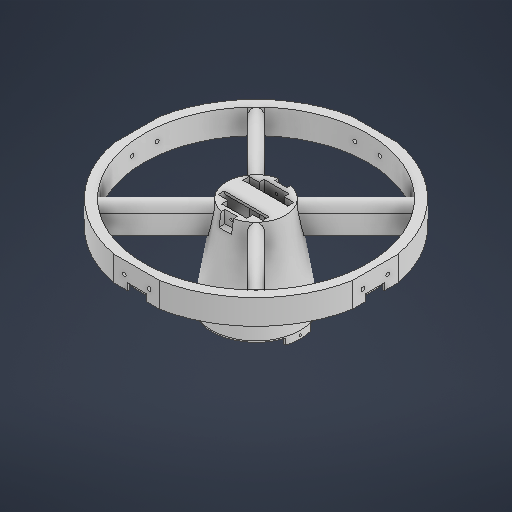
# Autodesk Inventor part: 004-002
Saved by Autodesk Inventor 2026 (Build 300175000, 175)
## iProperties
Created: 2026-04-19
Part Number: 004-002
Material: Ogólny
Document SubType Name: Modeling
Designer: Patryk Lombardo
Density: 1 g/cm^3
Appearance: Domyślna
Author: Patryk Lombardo
Autodesk Inventor part; units mm, degrees
ref_plane "YZ Plane" through (0, 0, 0) normal (1, 0, 0) x (0, 1, 0)
ref_plane "XZ Plane" through (0, 0, 0) normal (0, 1, 0) x (-1, 0, 0)
sketch "Szkic1" plane through (0, 0, 0) normal (0, 1, 0) x (-1, 0, 0)
  circle A0 centre (0, 0) radius 35.5
  dimension "d0" = 71
  constraints: 1 centre point, 1 coincident
  measures "d0" diameter of A0
extrude "Wyciągnięcie proste1" add sketch "Szkic1" against normal blind 1
ref_plane "Płaszczyzna konstrukcyjna1" through (0, 74, 0) normal (0, 1, 0) x (1, 0, 0)
sketch "Szkic2" plane through (0, 74, 0) normal (0, 1, 0) x (1, 0, 0)
  circle A0 centre (0, 0) radius 23.5
  line L0 (-18, 0) -> (18, 0) construction
  line L1 (0, -12.5) -> (0, 12.5) construction
  line L2 (18, 12.5) -> (18, -12.5) construction
  line L3 (-18, 12.5) -> (-18, -12.5) construction
  line L4 (-18, 12.5) -> (18, 12.5) construction
  line L5 (-18, -12.5) -> (18, -12.5) construction
  dimension "d4" = 47
  dimension "d5" = 36
  dimension "d6" = 25
  dimension "d7" = 12.5
  constraints: 12 end point, 4 midpoint, 3 vertical, 2 horizontal, 1 centre point, 1 coincident, 1 parallel
  measures "d4" diameter of A0
  measures "d5" distance of L0.start L0.end
  measures "d6" distance of L1.start L1.end
  measures "d7" distance between parallel lines of L4 L0
loft "Wyciągnięcie złożone1" add profiles "Szkic2" section 1 edges at (35.5, 0, 0)
sketch "Szkic3" plane through (0, 74, 0) normal (0, 1, 0) x (1, 0, 0)
  line L0 (-18, 0) -> (18, 0) construction
  line L1 (0, 12.5) -> (0, -12.5) construction
  line L2 (18, 12.5) -> (18, -12.5)
  line L3 (-18, 12.5) -> (-18, -12.5)
  line L4 (-18, 12.5) -> (18, 12.5)
  line L5 (-18, -12.5) -> (18, -12.5)
  line L6 (0, 12.5) -> (0, 16.5) construction
  line L7 (10, 16.5) -> (-10, 16.5)
  line L8 (-10, 16.5) -> (-10, 12.5)
  line L9 (10, 16.5) -> (10, 12.5)
  line L10 (0, -12.5) -> (0, -17.5) construction
  line L11 (-10, -17.5) -> (10, -17.5)
  line L12 (-10, -17.5) -> (-10, -12.5)
  line L13 (10, -17.5) -> (10, -12.5)
  point P0 (0, 0)
  dimension "d12" = 36
  dimension "d13" = 25
  dimension "d14" = 12.5
  dimension "d15" = 4
  dimension "d16" = 20
  dimension "d17" = 5
  dimension "d18" = 20
  constraints: 28 end point, 6 midpoint, 6 vertical, 4 perpendicular, 4 point on line, 3 horizontal, 1 parallel
  measures "d12" distance of L0.start L0.end
  measures "d13" distance of L1.start L1.end
  measures "d14" distance between parallel lines of L4 L0
  measures "d15" distance of L1.start L6.end
  measures "d16" distance of L7.start L7.end
  measures "d17" distance of L1.end L10.end
  measures "d18" distance of L11.start L11.end
extrude "Wyciągnięcie proste2" cut sketch "Szkic3" against normal through all
sketch "Szkic4" plane through (0, 74, 0) normal (0, 1, 0) x (1, 0, 0)
  line L0 (18, 0) -> (-18, 0) construction
  line L1 (-18, -7.5) -> (-18, 7.5)
  line L2 (18, -7.5) -> (18, 7.5)
  line L3 (-18, 7.5) -> (18, 7.5)
  line L4 (-18, -7.5) -> (18, -7.5)
  point P0 (0, 0)
  dimension "d21" = 36
  dimension "d22" = 15
  constraints: 10 end point, 3 midpoint, 2 horizontal, 2 vertical, 1 parallel
  measures "d21" distance of L0.start L0.end
  measures "d22" distance of L1.start L1.end
extrude "Wyciągnięcie proste3" add sketch "Szkic4" against normal blind 2
sketch "Szkic6" plane through (0, -1, 0) normal (0, -1, 0) x (1, 0, 0)
  line L0 (-19.5, 0) -> (19.5, 0) construction
  line L1 (0, 14) -> (0, -14) construction
  line L2 (19.5, 14.5) -> (19.5, -14.5)
  line L3 (-19.5, 14.5) -> (-19.5, -14.5)
  line L4 (-19.5, 14.5) -> (19.5, 14.5)
  line L5 (-19.5, -14.5) -> (19.5, -14.5)
  line L6 (0, 14) -> (0, 19) construction
  line L7 (12, 19) -> (-12, 19)
  line L8 (-12, 19) -> (-12, 14.5)
  line L9 (12, 19) -> (12, 14.5)
  line L10 (0, -14) -> (0, -19) construction
  line L11 (-12, -19) -> (12, -19)
  line L12 (-12, -19) -> (-12, -14.5)
  line L13 (12, -19) -> (12, -14.5)
  circle A0 centre (0, 0) radius 31
  dimension "d25" = 39
  dimension "d26" = 28
  dimension "d27" = 14.5
  dimension "d28" = 5
  dimension "d29" = 24
  dimension "d30" = 5
  dimension "d31" = 24
  dimension "d32" = 62
  constraints: 28 end point, 6 midpoint, 6 vertical, 4 perpendicular, 4 point on line, 3 horizontal, 2 coincident, 1 centre point, 1 parallel
  measures "d25" distance of L0.start L0.end
  measures "d26" distance of L1.start L1.end
  measures "d27" distance between parallel lines of L4 L0
  measures "d28" distance of L1.start L6.end
  measures "d29" distance of L7.start L7.end
  measures "d30" distance of L1.end L10.end
  measures "d31" distance of L11.start L11.end
  measures "d32" diameter of A0
extrude "Wyciągnięcie proste4" cut sketch "Szkic6" against normal blind 18
sketch "Szkic7" plane through (0, -1, 0) normal (0, -1, 0) x (1, 0, 0)
  line L0 (32, 0) -> (-32, 0) construction
  circle A0 centre (0, 0) radius 35.5
  line L1 (-32, -10) -> (-32, 10)
  line L2 (32, -10) -> (32, 10)
  line L3 (32, -10) -> (34.0624, -10)
  line L4 (32, 10) -> (34.0624, 10)
  line L5 (-32, -10) -> (-34.0624, -10)
  line L6 (-32, 10) -> (-34.0624, 10)
  dimension "d35" = 64
  dimension "d36" = 71
  dimension "d37" = 20
  dimension "d38" = 20
  constraints: 14 end point, 4 coincident, 4 horizontal, 4 point on circle, 3 midpoint, 2 vertical, 1 centre point, 1 parallel
  measures "d35" distance of L0.start L0.end
  measures "d36" diameter of A0
  measures "d37" distance of L1.start L1.end
  measures "d38" distance of L2.start L2.end
extrude "Wyciągnięcie proste5" add sketch "Szkic7" along normal blind 5 contours A0 L3 L2 L4 | L6 L1 L5 A0
sketch "Szkic8" plane through (32, -1, -10) normal (-1, 0, 0) x (0, 0, 1)
  line L0 (10, 1) -> (10, -2.5) construction
  circle A0 centre (10, -2.5) radius 1
  dimension "d41" = 3.5
  dimension "d42" = 2
  constraints: 2 end point, 1 centre point, 1 coincident, 1 vertical
  measures "d41" distance of L0.start L0.end
  measures "d42" diameter of A0
extrude "Wyciągnięcie proste6" cut sketch "Szkic8" along normal through all both and the other way through all
sketch "Szkic9" plane through (0, 74, 0) normal (0, 1, 0) x (1, 0, 0)
  circle A0 centre (0, 0) radius 23.5
  line L0 (0, -20) -> (0, 20) construction
  line L1 (-5, 20) -> (5, 20)
  line L2 (-5, -20) -> (5, -20)
  line L3 (5, 20) -> (5, 30)
  line L4 (5, -20) -> (5, -30)
  line L5 (-5, -20) -> (-5, -30)
  line L6 (-5, -30) -> (5, -30)
  line L7 (-5, 20) -> (-5, 30)
  line L8 (-5, 30) -> (5, 30)
  dimension "d45" = 47
  dimension "d46" = 40
  dimension "d47" = 10
  dimension "d48" = 10
  dimension "d49" = 10
  dimension "d50" = 10
  constraints: 18 end point, 4 vertical, 3 midpoint, 2 horizontal, 2 perpendicular, 1 centre point, 1 coincident, 1 point on line
  measures "d45" diameter of A0
  measures "d46" distance of L0.start L0.end
  measures "d47" distance of L2.start L2.end
  measures "d48" distance of L1.start L1.end
  measures "d49" distance of L1.end L3.end
  measures "d50" distance of L2.end L4.end
extrude "Wyciągnięcie proste7" cut sketch "Szkic9" against normal blind 10 contours L3 L1 L7 A0 | A0 L7 L8 L3 | L4 L6 L5 A0 | A0 L5 L2 L4
sketch "Szkic10" plane through (5, 74, -20) normal (0, 0, -1) x (-1, 0, 0)
  line L0 (0, 0) -> (5, 0) construction
  line L1 (5, 0) -> (5, -5) construction
  circle A0 centre (5, -5) radius 1
  point P0 (5, -74)
  dimension "d53" = 5
  dimension "d54" = 5
  dimension "d55" = 0
  dimension "d56" = 74
  dimension "d57" = 2
  constraints: 4 end point, 1 centre point, 1 coincident, 1 horizontal, 1 perpendicular
  measures "d53" distance of L0.start L0.end
  measures "d54" distance of L0.end L1.end
  measures "d55" distance from line of point (5, -74) L1
  measures "d56" distance from line of point (5, -74) L0
  measures "d57" diameter of A0
extrude "Wyciągnięcie proste8" cut sketch "Szkic10" against normal through all
sketch "Szkic11" plane through (-5, 74, 20) normal (0, 1, 0) x (1, 0, 0)
  circle A0 centre (5, 20) radius 90
  circle A1 centre (5, 20) radius 97.5
  line L0 (5, 20) -> (5, -75.75) construction
  line L1 (-13.3899, -75.75) -> (23.3899, -75.75)
  line L2 (5, 20) -> (100.75, 20) construction
  line L3 (100.75, 1.6101) -> (100.75, 38.3899)
  line L4 (5, 20) -> (5, 115.75) construction
  line L5 (23.3899, 115.75) -> (-13.3899, 115.75)
  line L6 (5, 20) -> (-90.75, 20) construction
  line L7 (-90.75, 38.3899) -> (-90.75, 1.6101)
  line L8 (5, 20) -> (68.6396, 83.6396) construction
  line L9 (64.9467, 87.1296) -> (72.1296, 79.9467)
  line L10 (5, 20) -> (-58.6396, 83.6396) construction
  line L11 (-62.1296, 79.9467) -> (-54.9467, 87.1296)
  line L12 (5, 20) -> (-58.6396, -43.6396) construction
  line L13 (-54.9467, -47.1296) -> (-62.1296, -39.9467)
  line L14 (5, 20) -> (68.6396, -43.6396) construction
  line L15 (72.1296, -39.9467) -> (64.9467, -47.1296)
  point P0 (-93.9108, 38.2483)
  point P1 (-93.9108, 1.4686)
  point P2 (-16.5506, -75.8915)
  point P3 (97.5892, 1.4686)
  point P4 (97.5892, 38.2483)
  point P5 (20.2291, 115.6085)
  point P6 (-16.5506, 115.6085)
  point P7 (68.5382, 83.5382)
  point P8 (-58.5382, 83.5382)
  point P9 (-58.5382, -43.5382)
  point P10 (68.5382, -43.5382)
  point P11 (-90.75, 1.6101)
  point P12 (-13.3899, -75.75)
  point P13 (-13.3899, 115.75)
  dimension "d63" = 195
  dimension "d62" = 180
  dimension "d64" = 95.75
  dimension "d65" = 360
  dimension "d66" = 45
  dimension "d67" = 10.1581
  dimension "d70" = 360
  constraints: 32 end point, 4 point on line, 3 coincident, 2 midpoint, 2 point on circle, 1 centre point, 1 horizontal, 1 perpendicular, 1 vertical, 57 other
  measures "d62" diameter of A0
  measures "d64" distance of L0.start L0.end
  measures "d66" angle of L4 L8
  measures "d67" distance of L9.start L9.end
extrude "Wyciągnięcie proste9" add sketch "Szkic11" against normal blind 20 contours L9 A0 | A0 L15 | L11 A0 | A0 L13 | L3 A1 L1 L7 L5
sketch "Szkic13" plane through (-5, 74, 20) normal (0, 1, 0) x (1, 0, 0)
  line L0 (5, 20) -> (5, 10) construction
  line L1 (5, 10) -> (5, 0) construction
  line L2 (5, 20) -> (5, 27) construction
  line L3 (10, 20) -> (0, 20) construction
  ellipse E0 centre (5, 20) end of major axis (0, 20) minor radius 7 (10, 20) -> (0, 20) ccw
  ellipse E1 centre (5, 20) end of major axis (0, 20) minor radius 20 (0, 20) -> (10, 20) ccw
  line L4 (2.25, 10) -> (7.75, 10)
  line L5 (7.75, 10) -> (7.75, 3.2967)
  line L6 (2.25, 10) -> (2.25, 3.2967)
  dimension "d80" = 10
  dimension "d81" = 7
  dimension "d82" = 10
  dimension "d83" = 10
  dimension "d84" = 5.5
  constraints: 14 end point, 4 horizontal, 4 vertical, 2 coincident, 2 midpoint, 1 point on line, 12 other
  measures "d80" distance of L3.end L3.start
  measures "d81" distance of L0.start L2.end
  measures "d82" distance of L0.end L1.end
  measures "d83" distance of L0.start L0.end
  measures "d84" distance of L4.start L4.end
sketch "Szkic14" plane through (59.9467, 54, -67.1296) normal (-0.7071068, 0, 0.7071068) x (0.7071068, 0, 0.7071068)
  line L0 (5.0791, 12.9138) -> (5.0791, 2.9138) construction
  line L1 (5.0791, 2.9138) -> (5.0791, -7.0862) construction
  line L2 (5.0791, 12.9138) -> (5.0791, 19.9138) construction
  line L3 (10.0791, 12.9138) -> (0.0791, 12.9138) construction
  ellipse E0 centre (5.0791, 12.9138) end of major axis (0.0791, 12.9138) minor radius 7 (10.0791, 12.9138) -> (0.0791, 12.9138) ccw
  ellipse E1 centre (5.0791, 12.9138) end of major axis (0.0791, 12.9138) minor radius 20 (0.0791, 12.9138) -> (10.0791, 12.9138) ccw
  line L4 (2.3291, 2.9138) -> (7.8291, 2.9138)
  line L5 (7.8291, 2.9138) -> (7.8291, -3.7895)
  line L6 (2.3291, 2.9138) -> (2.3291, -3.7895)
  point P0 (5.0791, -54)
  dimension "d85" = 10
  dimension "d86" = 7
  dimension "d87" = 10
  dimension "d88" = 10
  dimension "d89" = 5.5
  dimension "d90" = 2.75
  dimension "d91" = 66.9138
  constraints: 14 end point, 4 horizontal, 4 vertical, 2 coincident, 2 midpoint, 1 point on line, 12 other
  measures "d85" distance of L3.end L3.start
  measures "d86" distance of L0.start L2.end
  measures "d87" distance of L0.end L1.end
  measures "d88" distance of L0.start L0.end
  measures "d89" distance of L4.start L4.end
  measures "d90" distance from line of point (5.079, -54) L5
  measures "d91" distance from line of point (5.079, -54) L3
extrude "Wyciągnięcie proste10" add sketch "Szkic14" along normal up to surface contours E1 L5 L4 L6 E0
pattern_circular "Szyk kołowy1" count 4 over 360 about axis through (0, 0, 0) along (0, 1, 0) of "Wyciągnięcie proste10"
sketch "Szkic15" plane through (-5, 54, 20) normal (0, -1, 0) x (1, 0, 0)
  circle A0 centre (5, -20) radius 91.5
  circle A1 centre (5, -20) radius 94.5
  line L0 (5, -20) -> (-86.5, -20) construction
  line L1 (-86.5, -27.5) -> (-86.5, -12.5)
  line L2 (-86.5, -27.5) -> (-92.5, -27.5)
  line L3 (-92.5, -27.5) -> (-92.5, -12.5)
  line L4 (-92.5, -12.5) -> (-86.5, -12.5)
  line L5 (5, -20) -> (5, -111.5) construction
  line L6 (12.5, -111.5) -> (-2.5, -111.5)
  line L7 (12.5, -111.5) -> (12.5, -117.5)
  line L8 (12.5, -117.5) -> (-2.5, -117.5)
  line L9 (-2.5, -117.5) -> (-2.5, -111.5)
  line L10 (5, -20) -> (96.5, -20) construction
  line L11 (96.5, -12.5) -> (96.5, -27.5)
  line L12 (96.5, -12.5) -> (102.5, -12.5)
  line L13 (102.5, -12.5) -> (102.5, -27.5)
  line L14 (102.5, -27.5) -> (96.5, -27.5)
  line L15 (5, -20) -> (5, 71.5) construction
  line L16 (-2.5, 71.5) -> (12.5, 71.5)
  line L17 (-2.5, 71.5) -> (-2.5, 77.5)
  line L18 (-2.5, 77.5) -> (12.5, 77.5)
  line L19 (12.5, 77.5) -> (12.5, 71.5)
  circle A2 centre (5, -20) radius 35.5
  line L20 (5, -20) -> (-20.1023, -45.1023) construction
  line L21 (-2.955, -31.844) -> (-6.844, -27.955)
  line L22 (-6.844, -27.955) -> (-21.9714, -43.0823)
  line L23 (-2.955, -31.844) -> (-18.0823, -46.9714)
  line L24 (5, -20) -> (30.1023, -45.1023) construction
  line L25 (16.844, -27.955) -> (12.955, -31.844)
  line L26 (12.955, -31.844) -> (28.0823, -46.9714)
  line L27 (16.844, -27.955) -> (31.9714, -43.0823)
  line L28 (5, -20) -> (30.1023, 5.1023) construction
  line L29 (12.955, -8.156) -> (16.844, -12.045)
  line L30 (16.844, -12.045) -> (31.9714, 3.0823)
  line L31 (12.955, -8.156) -> (28.0823, 6.9714)
  line L32 (5, -20) -> (-20.1023, 5.1023) construction
  line L33 (-6.844, -12.045) -> (-2.955, -8.156)
  line L34 (-2.955, -8.156) -> (-18.0823, 6.9714)
  line L35 (-6.844, -12.045) -> (-21.9714, 3.0823)
  line L36 (-6.6295, -4.4814) -> (16.6295, -4.4814)
  line L37 (-6.6295, -35.5186) -> (16.6295, -35.5186)
  line L38 (-6.6295, -4.4814) -> (-6.6295, -35.5186)
  line L39 (16.6295, -4.4814) -> (16.6295, -35.5186)
  point P0 (-4.8995, -29.8995)
  point P1 (14.8995, -29.8995)
  point P2 (14.8995, -10.1005)
  point P3 (-4.8995, -10.1005)
  point P4 (-89.2019, -12.5)
  point P5 (-89.2019, -27.5)
  point P6 (-2.5, -114.2019)
  point P7 (12.5, -114.2019)
  point P8 (99.2019, -27.5)
  point P9 (99.2019, -12.5)
  point P10 (12.5, 74.2019)
  point P11 (-2.5, 74.2019)
  point P12 (-21.9714, 3.0823)
  point P13 (5, -4.4814)
  point P14 (16.6295, -28.1694)
  point P15 (16.6295, -11.8306)
  point P16 (-6.6295, -4.4814)
  point P17 (-6.6295, -11.8306)
  point P18 (-6.6295, -28.1694)
  dimension "d97" = 183
  dimension "d98" = 189
  dimension "d99" = 15
  dimension "d100" = 6
  dimension "d103" = 360
  dimension "d105" = 71
  dimension "d106" = 45
  dimension "d107" = 5.5
  dimension "d108" = 14
  dimension "d109" = 21.3933
  dimension "d112" = 360
  dimension "d116" = 23.2591
  dimension "d117" = 23.2591
  constraints: 80 end point, 8 point on line, 4 perpendicular, 3 coincident, 3 horizontal, 3 midpoint, 3 point on circle, 2 centre point, 2 vertical, 1 horizontal alignment, 1 parallel, 92 other
  measures "d98" diameter of A1
  measures "d99" distance of L1.start L1.end
  measures "d100" distance of L1.start L2.end
  measures "d105" diameter of A2
  measures "d106" angle of L5 L20
  measures "d107" distance of L21.start L21.end
  measures "d108" distance of point (-4.899, -29.899) point (5, -20)
  measures "d109" distance of L21.end L22.end
  measures "d116" distance of L37.start L37.end
  measures "d117" distance of L36.start L36.end
extrude "Wyciągnięcie proste11" cut sketch "Szkic15" against normal blind 5.5 contours L11 L14 A1 L7 L6 A0 | A0 L16 L19 A1 L12 L11 | L11 L12 A1 L14 | A0 L1 L4 A1 L17 L16 | L16 L17 A1 L19 | L6 L9 A1 L2 L1 A0 | L6 L7 A1 L9 | L1 L2 A1 L4 | L12 L13 L14 A1 | L17 L18 L19 A1 | L7 L8 L9 A1 | L2 L3 L4 A1 | L30 L29 L39 L31 A2 | A2 L26 L39 L25 L27 | L34 L38 L33 L35 A2 | L39 L29 L31 | L31 L29 L39 L25 L26 L37 L23 L21 L38 L33 L34 L36 | A2 L22 L21 L38 L23 | L26 L25 L39 | L34 L33 L38 | L38 L21 L23
sketch "Szkic16" plane through (95.75, 74, 18.3899) normal (1, 0, 0) x (0, 0, -1)
  line L0 (0, 0) -> (18.3899, 0) construction
  line L1 (18.3899, 0) -> (18.3899, -10) construction
  line L2 (8.3899, -10) -> (28.3899, -10) construction
  circle A0 centre (28.3899, -10) radius 1.5
  circle A1 centre (8.3899, -10) radius 1.5
  point P0 (18.3899, -74)
  dimension "d118" = 18.3899
  dimension "d119" = 74
  dimension "d120" = 74
  dimension "d121" = 10
  dimension "d122" = 20
  dimension "d123" = 3
  dimension "d124" = 3
  constraints: 6 end point, 2 centre point, 2 coincident, 2 horizontal, 1 midpoint, 1 vertical
  measures "d118" distance of L0.start L0.end
  measures "d119" distance from line of point (18.39, -74) L0
  measures "d120" distance of point (18.39, -74) L0.end
  measures "d121" distance of L0.end L1.end
  measures "d122" distance of L2.start L2.end
  measures "d123" diameter of A0
  measures "d124" diameter of A1
extrude "Wyciągnięcie proste12" cut sketch "Szkic16" against normal up to surface
pattern_circular "Szyk kołowy2" count 4 over 360 about axis through (0, 0, 0) along (0, 1, 0) of "Wyciągnięcie proste12"
